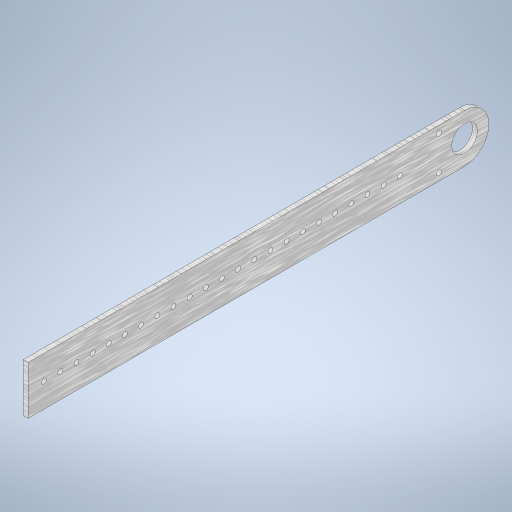
# Autodesk Inventor part: shoulder1_upper_plate
Saved by Autodesk Inventor 2024 (Build 280153000, 153)
## iProperties
Company: 細田研究室
Created: 2025-06-07
Part Number: shoulder1_upper_plate
Material: アルミニウム 5052
Document SubType Name: Modeling
Designer: HosodaLab2
Density: 2.68 g/cm^3
Appearance: サテン - ブラシ仕上げ 重厚
Mass: 70.367 g
Surface Area: 200.69 cm^2
Volume: 26.0618 cm^3
Stock Number: 1
個数: 1
Author: HosodaLab2
Autodesk Inventor part; units mm, degrees
ref_plane "YZ Plane" through (0, 0, 0) normal (1, 0, 0) x (0, 1, 0)
ref_plane "XZ Plane" through (0, 0, 0) normal (0, 1, 0) x (-1, 0, 0)
ref_plane "XY Plane" through (0, 0, 0) normal (0, 0, 1) x (1, 0, 0)
sketch "スケッチ1" plane through (0, 0, 0) normal (0, 1, 0) x (-1, 0, 0)
  line L0 (0, 0) -> (-287.5, 0)
  line L1 (-287.5, 0) -> (-287.5, -30)
  line L2 (-287.5, -30) -> (0, -30)
  line L3 (0, -30) -> (0, 0)
  arc A0 (-17.5, -30) -> (-17.5, 0) centre (-17.5, -15) ccw
  dimension "d0" = 287.5
  dimension "d1" = 30
  dimension "d43" = 17.5
  constraints: 8 end point, 2 parallel, 2 point on circle, 2 point on line, 2 tangent, 1 centre point, 1 horizontal, 1 perpendicular
  measures "d0" distance of L2.end L1.end
  measures "d1" distance of L1.end L0.end
  measures "d43" distance from line of L3 A0.centre
extrude "押し出し1" add sketch "スケッチ1" along normal blind 3 contours A0 L2 L1 L0
sketch "スケッチ2" plane through (0, 3, 0) normal (0, 1, 0) x (1, 0, 0)
  arc A0 (17.5, 30) -> (17.5, 0) centre (17.5, 15) ccw projected
  line L0 (287.5, 30) -> (17.5, 30) projected
  point P0 (0, 0)
  point P1 (2.5, 15)
  constraints: 1 coincident, 1 point on circle
hole "穴1" at (17.5, 3, -15) direction (0, -1, 0) diameter 16 end through all
sketch "スケッチ3" plane through (0, 3, 0) normal (0, 1, 0) x (1, 0, 0)
  line L0 (287.5, 0) -> (287.5, 30) projected
  arc A0 (17.5, 30) -> (17.5, 0) centre (17.5, 15) ccw construction
  line L1 (17.5, 15) -> (287.5, 15) construction
  line L2 (287.5, 0) -> (287.5, 30) construction
  point P0 (0, 0)
  point P1 (57.5, 15)
  point P2 (67.5, 15)
  point P3 (77.5, 15)
  point P4 (87.5, 15)
  point P5 (97.5, 15)
  point P6 (107.5, 15)
  point P7 (117.5, 15)
  point P8 (127.5, 15)
  point P9 (137.5, 15)
  point P10 (147.5, 15)
  point P11 (157.5, 15)
  point P12 (167.5, 15)
  point P13 (177.5, 15)
  point P14 (187.5, 15)
  point P15 (197.5, 15)
  point P16 (207.5, 15)
  point P17 (217.5, 15)
  point P18 (227.5, 15)
  point P19 (237.5, 15)
  point P20 (247.5, 15)
  point P21 (257.5, 15)
  point P22 (267.5, 15)
  point P23 (277.5, 15)
  dimension "d108" = 40
  dimension "d111" = 10
  constraints: 2 end point, 1 horizontal, 1 midpoint, 1 perpendicular, 1 point on line, 22 other
  measures "d108" distance of point (57.5, 15) L1.start
  measures "d111" distance of point (57.5, 15) point (67.5, 15)
sketch "スケッチ8" plane through (0, 3, 0) normal (0, 1, 0) x (1, 0, 0)
  arc A0 (17.5, 30) -> (17.5, 0) centre (17.5, 15) ccw projected
  line L0 (2.5, 15) -> (40.1182, 15)
  line L1 (17.5, 0) -> (287.5, 0) projected
  line L2 (2.5, 15) -> (302.5, 15) construction
  circle A1 centre (17.5, 15) radius 8 construction
  point P0 (0, 0)
  point P1 (33.3, 4.5)
  point P2 (33.3, 25.5)
  dimension "d85" = 10.5
  dimension "d86" = 10.5
  dimension "d123" = 15.8
  dimension "d124" = 15.8
  constraints: 4 end point, 2 horizontal, 1 point on circle
  measures "d85" distance from line of point (33.3, 4.5) L0
  measures "d86" distance from line of point (33.3, 25.5) L0
  measures "d123" horizontal distance of point (33.3, 4.5) A1.centre
  measures "d124" horizontal distance of point (33.3, 25.5) A1.centre
hole "穴6" at (33.3, 3, -4.5) at (33.3, 3, -25.5) direction (0, -1, 0) diameter 3.3 end through all
hole "穴7" at (57.5, 3, -15) at (67.5, 3, -15) at (77.5, 3, -15) at (87.5, 3, -15) at (97.5, 3, -15) at (107.5, 3, -15) at (117.5, 3, -15) at (127.5, 3, -15) at (137.5, 3, -15) at (147.5, 3, -15) at (157.5, 3, -15) at (167.5, 3, -15) at (177.5, 3, -15) at (187.5, 3, -15) at (197.5, 3, -15) at (207.5, 3, -15) at (217.5, 3, -15) at (227.5, 3, -15) at (237.5, 3, -15) at (247.5, 3, -15) at (257.5, 3, -15) at (267.5, 3, -15) at (277.5, 3, -15) direction (0, -1, 0) diameter 3.2 end through all
